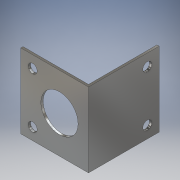
# Autodesk Inventor part: ks dianteiro F
Saved by Autodesk Inventor 2019 (Build 230136000, 136)
## iProperties
Created: 2020-06-04
Part Number: ks dianteiro F
Material: Aço cromado
Document SubType Name: Modeling
Designer: eliane
Density: 7.85 g/cm^3
Appearance: Cromado - Polido
Author: eliane
Autodesk Inventor part; units mm, degrees
ref_plane "YZ Plane" through (0, 0, 0) normal (1, 0, 0) x (0, 1, 0)
ref_plane "XZ Plane" through (0, 0, 0) normal (0, 1, 0) x (-1, 0, 0)
ref_plane "XY Plane" through (0, 0, 0) normal (0, 0, 1) x (1, 0, 0)
sketch "Esboço1" plane through (0, 0, 0) normal (0, 0, 1) x (1, 0, 0)
  circle A0 centre (0, 0) radius 12.5
  line L0 (0, 0) -> (18, 0) construction
  line L1 (0, 0) -> (-26, 0) construction
  line L2 (0, 0) -> (0, 25) construction
  line L3 (0, 0) -> (0, -25) construction
  line L4 (-26, 25) -> (18, 25)
  line L5 (18, 25) -> (18, -25)
  line L6 (18, -25) -> (-26, -25)
  line L7 (-26, -25) -> (-26, 25)
  line L8 (-26, 25) -> (-18, 25) construction
  line L9 (-18, 25) -> (-18, 17) construction
  circle A1 centre (-18, 17) radius 3
  line L10 (-26, -25) -> (-18, -25) construction
  line L11 (-18, -25) -> (-18, -17) construction
  circle A2 centre (-18, -17) radius 3
  dimension "d0" = 25
  dimension "d1" = 18
  dimension "d2" = 26
  dimension "d3" = 25
  dimension "d4" = 25
  dimension "d5" = 8
  dimension "d6" = 8
  dimension "d7" = 6
  dimension "d8" = 8
  dimension "d9" = 8
  dimension "d10" = 6
  constraints: 24 end point, 3 centre point, 3 coincident, 3 horizontal, 3 perpendicular, 2 parallel, 2 point on line, 2 vertical
  measures "d0" diameter of A0
  measures "d1" distance of L0.start L0.end
  measures "d2" distance of L0.start L1.end
  measures "d3" distance of L0.start L2.end
  measures "d4" distance of L0.start L3.end
  measures "d5" distance of L4.start L8.end
  measures "d6" distance of L8.end L9.end
  measures "d7" diameter of A1
  measures "d8" distance of L6.end L10.end
  measures "d9" distance of L10.end L11.end
  measures "d10" diameter of A2
extrude "Extrusão1" add sketch "Esboço1" along normal blind 1.5
sketch "Esboço2" plane through (18, -25, 0) normal (1, 0, 0) x (0, 0, -1)
  line L0 (-1.5, 50) -> (46, 50)
  line L1 (46, 50) -> (46, 0)
  line L2 (46, 0) -> (-1.5, 0)
  line L3 (-1.5, 0) -> (-1.5, 50)
  line L4 (46, 50) -> (38, 50) construction
  line L5 (38, 50) -> (38, 42) construction
  circle A0 centre (38, 42) radius 3
  line L6 (46, 0) -> (38, 0) construction
  line L7 (38, 0) -> (38, 8) construction
  circle A1 centre (38, 8) radius 3
  point P0 (0, 25)
  dimension "d13" = 47.5
  dimension "d14" = 50
  dimension "d15" = 8
  dimension "d16" = 8
  dimension "d17" = 6
  dimension "d18" = 8
  dimension "d19" = 8
  dimension "d20" = 6
  constraints: 16 end point, 3 perpendicular, 2 centre point, 2 coincident, 2 parallel, 2 point on line, 1 horizontal
  measures "d13" distance of L1.end L2.end
  measures "d14" distance of L0.end L1.end
  measures "d15" distance of L0.end L4.end
  measures "d16" distance of L4.end L5.end
  measures "d17" diameter of A0
  measures "d18" distance of L1.end L6.end
  measures "d19" distance of L6.end L7.end
  measures "d20" diameter of A1
extrude "Extrusão2" add sketch "Esboço2" along normal blind 1.5
